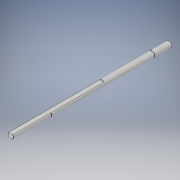
# Autodesk Inventor part: walek
Saved by Autodesk Inventor 2019 (Build 230136000, 136)
## iProperties
Created: 2020-05-17
Part Number: walek
Material: Generic
Document SubType Name: Modeling
Designer: estee
Density: 1 g/cm^3
Appearance: Default
Author: estee
Autodesk Inventor part; units mm, degrees
ref_plane "YZ Plane" through (0, 0, 0) normal (1, 0, 0) x (0, 1, 0)
ref_plane "XZ Plane" through (0, 0, 0) normal (0, 1, 0) x (-1, 0, 0)
ref_plane "XY Plane" through (0, 0, 0) normal (0, 0, 1) x (1, 0, 0)
sketch "Sketch1" plane through (0, 0, 0) normal (0, 0, 1) x (1, 0, 0)
  circle A0 centre (0, 0) radius 6
  dimension "d0" = 12
  constraints: 1 centre point, 1 coincident
  measures "d0" diameter of A0
extrude "Extrusion1" add sketch "Sketch1" along normal blind 336.5
chamfer "Chamfer1" distance 0.5 angle 45 2 edges at (-6, 0, 336.5) (-6, 0, 0)
sketch "Sketch2" plane through (0, 0, 336.5) normal (0, 0, 1) x (1, 0, 0)
  line L0 (-4.4614, 4) -> (4.4928, 4)
  point P0 (0, 0)
  dimension "d6" = 4
  constraints: 2 end point, 1 horizontal
  measures "d6" distance from line of L0 point (0, 0)
extrude "Extrusion2" cut sketch "Sketch2" against normal blind 193.6 fills toward (0.0157, 4.05) open curves L0
sketch "Szkic3" plane through (0, 0, 0) normal (1, 0, 0) x (0, 1, 0)
  line L0 (6.0582, 36.3) -> (5.8082, 36.3)
  line L1 (5.8082, 36.3) -> (5.8082, 37.3)
  line L2 (5.8082, 37.3) -> (6.0582, 37.3)
  line L3 (6.0582, 37.3) -> (6.0582, 36.3)
  line L4 (5.5, 0) -> (-5.5, 0) projected
  line L5 (0, -7.46) -> (0, 44.76) projected
  point P0 (0, 0)
  dimension "d16" = 36.3
  dimension "d17" = 1
  dimension "d18" = 0.25
  constraints: 8 end point, 2 parallel, 1 horizontal, 1 perpendicular
  measures "d16" distance between parallel lines of L4 L0
  measures "d17" distance of L2.end L0.start
  measures "d18" distance of L1.end L2.end
revolve "Obrót1" cut sketch "Szkic3" angle 360 about axis through (0, 0, -10) along (0, 0, 1)
sketch "Szkic4" plane through (0, 0, 0) normal (1, 0, 0) x (0, 1, 0)
  line L0 (-6, 37.3) -> (-6, 336) projected
  line L1 (-6, 256.2) -> (-5.75, 256.2)
  line L2 (-5.75, 256.2) -> (-5.75, 255.2)
  line L3 (-5.75, 255.2) -> (-6, 255.2)
  line L4 (-6, 255.2) -> (-6, 256.2)
  line L5 (-5.5, 336.5) -> (4, 336.5) projected
  line L6 (0, -50) -> (0, 300) projected
  point P0 (0, 0)
  dimension "d21" = 1
  dimension "d22" = 0.25
  dimension "d23" = 80.3
  constraints: 8 end point, 2 parallel, 1 horizontal, 1 perpendicular, 1 point on line
  measures "d21" distance between parallel lines of L3 L1
  measures "d22" distance between parallel lines of L0 L2
  measures "d23" distance between parallel lines of L5 L1
revolve "Obrót2" cut sketch "Szkic4" angle 360 about axis through (0, 0, -10) along (0, 0, 1)
body "Solid1"
